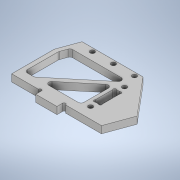
# Autodesk Inventor part: Trunk_lower_side_frame
Saved by Autodesk Inventor 2020.4 (Build 244396000, 396)
## iProperties
Created: 2022-01-02
Part Number: Trunk_lower_side_frame
Material: 一般
Document SubType Name: Modeling
Designer: Masato Kubotera
Density: 1 g/cm^3
Appearance: 既定
Mass: 14.6824 g
Surface Area: 92.1199 cm^2
Volume: 14.6824 cm^3
Description: A2017 T5
Author: Masato Kubotera
Autodesk Inventor part; units mm, degrees
ref_plane "YZ Plane" through (0, 0, 0) normal (1, 0, 0) x (0, 1, 0)
ref_plane "XZ Plane" through (0, 0, 0) normal (0, 1, 0) x (-1, 0, 0)
ref_plane "XY Plane" through (0, 0, 0) normal (0, 0, 1) x (1, 0, 0)
derived "Trunk_basis.ipt"
sketch "スケッチ1" plane through (0, 0, 0) normal (0, 1, 0) x (-1, 0, 0)
  line L0 (0, 22) -> (0, -143) construction
  circle A0 centre (5, 0) radius 10.5 construction
  line L1 (-7, 16) -> (36, 16) construction
  line L2 (36, 16) -> (36, -16) construction
  line L3 (36, -16) -> (-7, -16) construction
  line L4 (-7, -16) -> (-7, 16) construction
  line L5 (-7, 16) -> (36, -16) construction
  line L6 (36, 16) -> (-7, -16) construction
  line L7 (33, 13.5) -> (6, 13.5) construction
  line L8 (6, 13.5) -> (6, -13.5) construction
  line L9 (6, -13.5) -> (33, -13.5) construction
  line L10 (33, -13.5) -> (33, 13.5) construction
  line L11 (33, 13.5) -> (6, -13.5) construction
  line L12 (6, 13.5) -> (33, -13.5) construction
  line L13 (-7, 0) -> (36, 0) construction
  arc A1 (5, 16) -> (-7, 10.583) centre (5, 0) ccw construction
  line L14 (34.5651, -16.05) -> (5, -16.05) projected
  line L15 (5, 16.05) -> (34.5651, 16.05) projected
  line L16 (36.05, 14.5651) -> (36.05, -14.5651) projected
  line L17 (36.05, -16.05) -> (-7.05, 16.05) construction
  line L18 (-7.05, -16.05) -> (36.05, 16.05) construction
  arc A2 (5, 16.05) -> (-6.5314, 11.1638) centre (5, 0) ccw projected
  arc A3 (-6.5314, 11.1638) -> (-7.05, 9.8372) centre (-6.0721, 10.2196) ccw projected
  arc A4 (36.05, 14.5651) -> (34.5651, 16.05) centre (35.3075, 15.3075) ccw projected
  circle A5 centre (6, 13.5) radius 1.35 construction
  line L19 (19.5, 13.5) -> (19.5, -13.5) construction
  circle A6 centre (33, 13.5) radius 1.35 construction
  line L20 (-12, 22) -> (-17, 17) projected
  line L21 (-17, 17) -> (-17, -16) projected
  line L22 (-17, -16) -> (-28.5, -27.5) projected
  line L23 (-28.5, -27.5) -> (-28.5, -97) projected
  line L24 (54.5, -16) -> (54.5, 17) projected
  line L25 (54.5, 17) -> (49.5, 22) projected
  line L26 (49.5, 22) -> (-12, 22) projected
  line L27 (-28.5, -108.8772) -> (-28.5, -139) projected
  line L28 (-16, -138.9955) -> (-16, -99.5) construction
  line L29 (-16, -99.5) -> (16, -99.5) construction
  line L30 (16, -138.9955) -> (16, -99.5) construction
  line L31 (-7.5, -139) -> (-7.5, -143) projected
  line L32 (-7.5, -143) -> (7.5, -143) projected
  line L33 (7.5, -139) -> (7.5, -143) projected
  arc A7 (-7.5, -139) -> (-9.6, -139) centre (-8.55, -139) ccw projected
  arc A8 (9.6, -139) -> (7.5, -139) centre (8.55, -139) ccw projected
  line L34 (-22, -138.9955) -> (-22, -133) construction
  line L35 (-23.5, -133) -> (-20.5, -133) construction
  line L36 (-23.5, -133) -> (-23.5, -139) construction
  line L37 (-20.5, -133) -> (-20.5, -139) construction
  line L38 (-12, 22) -> (-7, 22) construction
  line L39 (-7, 22) -> (-7, -22) construction
  line L40 (-7, -22) -> (-12, -22) construction
  line L41 (-12, -22) -> (-12, 22) construction
  line L42 (-12, 22) -> (-7, -22) construction
  line L43 (-7, 22) -> (-12, -22) construction
  line L44 (-9.5, 22) -> (-9.5, -22) construction
  line L45 (-7, 0) -> (-12, 0) construction
  circle A9 centre (-9.5, 17.75) radius 1.6 projected
  line L46 (-12, 10) -> (-9.5, 10) construction
  line L47 (-9.5, 10) -> (-9.5, -10) construction
  line L48 (-9.5, -10) -> (-12, -10) construction
  line L49 (-12, -10) -> (-12, 10) construction
  line L50 (-12, 10) -> (-9.5, -10) construction
  line L51 (-9.5, 10) -> (-12, -10) construction
  line L52 (-9.45, 10.05) -> (-12.05, 10.05) projected
  line L53 (-12.05, 7.95) -> (-12.05, -7.95) projected
  line L54 (-12.05, -10.05) -> (-9.45, -10.05) projected
  line L55 (-9.45, -7.95) -> (-9.45, 7.95) projected
  line L56 (-9.45, 10.05) -> (-12.05, -10.05) construction
  line L57 (-12.05, 10.05) -> (-9.45, -10.05) construction
  arc A10 (-12.05, 10.05) -> (-12.05, 7.95) centre (-12.05, 9) ccw projected
  line L58 (-10.75, 10) -> (-10.75, -10) construction
  arc A11 (-9.45, 7.95) -> (-9.45, 10.05) centre (-9.45, 9) ccw projected
  circle A12 centre (-9.5, -17.75) radius 1.6 projected
  arc A13 (-12.05, -7.95) -> (-12.05, -10.05) centre (-12.05, -9) ccw projected
  arc A14 (-9.45, -10.05) -> (-9.45, -7.95) centre (-9.45, -9) ccw projected
  line L59 (36, 14.4) -> (44.5, 14.4) construction
  line L60 (44.5, 14.4) -> (44.5, -14.4) construction
  line L61 (36, -14.4) -> (44.5, -14.4) construction
  line L62 (46.95, 7.95) -> (46.95, -7.95) projected
  line L63 (49.5, 0) -> (44.5, 0) construction
  line L64 (44.5, 22) -> (49.5, 22) construction
  line L65 (49.55, -7.95) -> (49.55, 7.95) projected
  line L66 (48.25, 10) -> (48.25, -10) construction
  line L67 (49.5, 10) -> (47, -10) construction
  line L68 (49.5, -10) -> (47, -10) construction
  line L69 (49.5, 10) -> (49.5, -10) construction
  line L70 (47, 10) -> (49.5, -10) construction
  line L71 (46.95, -10.05) -> (49.55, -10.05) projected
  line L72 (46.95, 10.05) -> (49.55, -10.05) construction
  line L73 (49.55, 10.05) -> (46.95, -10.05) construction
  line L74 (49.5, -22) -> (44.5, -22) construction
  line L75 (44.5, 22) -> (49.5, -22) construction
  line L76 (49.5, 22) -> (49.5, -22) construction
  line L77 (49.5, 22) -> (44.5, -22) construction
  line L78 (47, 22) -> (47, -22) construction
  line L79 (44.5, -22) -> (44.5, 22) construction
  circle A15 centre (47, -17.75) radius 1.6 projected
  arc A16 (49.55, -10.05) -> (49.55, -7.95) centre (49.55, -9) ccw projected
  line L80 (47, -10) -> (47, 10) construction
  arc A17 (46.95, -7.95) -> (46.95, -10.05) centre (46.95, -9) ccw projected
  arc A18 (46.95, 10.05) -> (46.95, 7.95) centre (46.95, 9) ccw projected
  arc A19 (49.55, 7.95) -> (49.55, 10.05) centre (49.55, 9) ccw projected
  line L81 (47, 10) -> (49.5, 10) construction
  line L82 (49.55, 10.05) -> (46.95, 10.05) projected
  circle A20 centre (47, 17.75) radius 1.6 projected
  circle A21 centre (5, 0) radius 16 construction
  arc A22 (-6.5314, -11.1638) -> (5, -16.05) centre (5, 0) ccw projected
  arc A23 (-7.05, -9.8372) -> (-6.5314, -11.1638) centre (-6.0721, -10.2196) ccw projected
  arc A24 (34.5651, -16.05) -> (36.05, -14.5651) centre (35.3075, -15.3075) ccw projected
  line L83 (-7.05, -9.8372) -> (-7.05, 9.8372) projected
  line L84 (22, -138.9955) -> (22, -133) construction
  line L85 (23.5, -133) -> (23.5, -139) construction
  line L86 (20.5, -133) -> (20.5, -139) construction
  line L87 (23.5, -133) -> (20.5, -133) construction
  circle A25 centre (6, -13.5) radius 1.35 projected
  circle A26 centre (33, -13.5) radius 1.35 projected
  line L88 (188, -110.7642) -> (183, -110.7642) projected
  line L89 (183, -110.7642) -> (183, -167.2358) construction
  line L90 (183, -167.2358) -> (188, -167.2358) construction
  line L91 (188, -167.2358) -> (188, -110.7642) projected
  line L92 (188, -110.7642) -> (183, -167.2358) construction
  line L93 (183, -110.7642) -> (188, -167.2358) construction
  line L94 (22, -108.5) -> (56, -108.5) construction
  line L95 (56, -108.5) -> (56, -131.5) construction
  line L96 (56, -131.5) -> (22, -131.5) construction
  line L97 (22, -131.5) -> (22, -108.5) construction
  line L98 (22, -108.5) -> (56, -131.5) construction
  line L99 (56, -108.5) -> (22, -131.5) construction
  line L100 (22, -131.5) -> (52, -131.5) construction
  line L101 (52, -131.5) -> (52, -136.5) construction
  line L102 (52, -136.5) -> (22, -136.5) construction
  line L103 (22, -136.5) -> (22, -131.5) construction
  line L104 (22, -131.5) -> (52, -136.5) construction
  line L105 (52, -131.5) -> (22, -136.5) construction
  line L106 (-25.5, -131) -> (-25.5, -109.2298) projected
  line L107 (-8.2765, -133) -> (12.5, -133) projected
  line L108 (11.2211, -112.1814) -> (-9.5554, -129.4624) projected
  line L109 (22, -99.5) -> (17, -99.5) construction
  line L110 (17, -99.5) -> (17, -139) construction
  line L111 (17, -139) -> (22, -139) construction
  line L112 (22, -139) -> (22, -99.5) construction
  line L113 (22, -99.5) -> (17, -139) construction
  line L114 (17, -99.5) -> (22, -139) construction
  line L115 (19.5, -99.5) -> (19.5, -139) construction
  circle A27 centre (19.5, -107.25) radius 1.6 projected
  line L116 (17, -119.25) -> (22, -119.25) construction
  line L117 (-28.5, -139) -> (-28.5, -143) construction
  line L118 (-28.5, -143) -> (-7.5, -143) construction
  line L119 (28.5, -143) -> (7.5, -143) construction
  line L120 (28.5, -139) -> (28.5, -143) construction
  circle A28 centre (19.5, -131.25) radius 1.6 projected
  line L121 (17, -111.75) -> (22, -111.75) construction
  line L122 (17, -126.75) -> (22, -126.75) construction
  line L123 (39.4409, -150.6176) -> (61.7571, -150.6176) projected
  line L124 (63.242, -152.1025) -> (63.242, -179.9354) projected
  line L125 (61.7571, -181.4204) -> (39.4409, -181.4204) projected
  line L126 (37.9559, -179.9354) -> (37.9559, -152.1025) projected
  line L127 (37.9559, -150.6176) -> (63.242, -181.4204) construction
  line L128 (63.242, -150.6176) -> (37.9559, -181.4204) construction
  arc A29 (39.4409, -150.6176) -> (37.9559, -152.1025) centre (38.6984, -151.36) ccw projected
  line L129 (50.599, -150.6176) -> (50.599, -181.4204) construction
  line L130 (37.9559, -166.019) -> (63.242, -166.019) construction
  arc A30 (63.242, -152.1025) -> (61.7571, -150.6176) centre (62.4995, -151.36) ccw projected
  arc A31 (37.9559, -179.9354) -> (39.4409, -181.4204) centre (38.6984, -180.6779) ccw projected
  arc A32 (61.7571, -181.4204) -> (63.242, -179.9354) centre (62.4995, -180.6779) ccw projected
  arc A33 (18.4349, -111.7) -> (16.95, -113.1849) centre (17.6925, -112.4425) ccw projected
  line L131 (18.4349, -111.7) -> (20.5651, -111.7) projected
  arc A34 (22.05, -113.1849) -> (20.5651, -111.7) centre (21.3075, -112.4425) ccw projected
  line L132 (16.95, -125.3151) -> (16.95, -113.1849) projected
  line L133 (16.95, -119.25) -> (22.05, -119.25) construction
  arc A35 (16.95, -125.3151) -> (18.4349, -126.8) centre (17.6925, -126.0575) ccw projected
  line L134 (19.5, -111.7) -> (19.5, -126.8) construction
  line L135 (16.95, -111.7) -> (22.05, -126.8) construction
  line L136 (22.05, -111.7) -> (16.95, -126.8) construction
  line L137 (20.5651, -126.8) -> (18.4349, -126.8) projected
  line L138 (22.05, -113.1849) -> (22.05, -125.3151) projected
  arc A36 (20.5651, -126.8) -> (22.05, -125.3151) centre (21.3075, -126.0575) ccw projected
  line L139 (37, -131.5) -> (37, -136.5) construction
  line L140 (32, -131.5) -> (32, -136.5) construction
  line L141 (52, -134) -> (22, -134) projected
  circle A37 centre (27, -134) radius 1.6 projected
  arc A38 (42.05, -132.9349) -> (40.5651, -131.45) centre (41.3075, -132.1925) ccw projected
  arc A39 (33.4349, -131.45) -> (31.95, -132.9349) centre (32.6925, -132.1925) ccw projected
  line L142 (31.95, -134) -> (42.05, -134) construction
  line L143 (33.4349, -131.45) -> (40.5651, -131.45) projected
  line L144 (42.05, -132.9349) -> (42.05, -135.0651) projected
  line L145 (40.5651, -136.55) -> (33.4349, -136.55) projected
  line L146 (31.95, -135.0651) -> (31.95, -132.9349) projected
  line L147 (31.95, -131.45) -> (42.05, -136.55) construction
  line L148 (42.05, -131.45) -> (31.95, -136.55) construction
  line L149 (37, -131.45) -> (37, -136.55) construction
  arc A40 (31.95, -135.0651) -> (33.4349, -136.55) centre (32.6925, -135.8075) ccw projected
  arc A41 (40.5651, -136.55) -> (42.05, -135.0651) centre (41.3075, -135.8075) ccw projected
  line L150 (42, -131.5) -> (42, -136.5) construction
  circle A42 centre (47, -134) radius 1.6 projected
  line L151 (-23.6994, -103.9301) -> (-25.3794, -108.5458) projected
  line L152 (-23.5, -133) -> (-19.223, -133) projected
  line L153 (-17.9441, -132.5376) -> (13.7789, -106.1518) projected
  line L154 (-23.5, -22.5) -> (61, -22.5) construction
  line L155 (54.5, -16) -> (61, -22.5) projected
  line L156 (61, -22.5) -> (61, -89.4955) projected
  circle A43 centre (-13.5, -55) radius 1.75 projected
  line L157 (-16.5, -59) -> (49, -59) projected
  line L158 (51, -61) -> (51, -87.5) projected
  line L159 (49, -89.5) -> (-16.5, -89.5) projected
  line L160 (-18.5, -87.5) -> (-18.5, -61) projected
  line L161 (-18.5, -59) -> (51, -89.5) construction
  line L162 (51, -59) -> (-18.5, -89.5) construction
  line L163 (-16.5, -27.5) -> (49, -27.5) projected
  line L164 (51, -29.5) -> (51, -49) projected
  line L165 (49, -51) -> (-16.5, -51) projected
  line L166 (-18.5, -49) -> (-18.5, -29.5) projected
  line L167 (-18.5, -27.5) -> (51, -51) construction
  line L168 (51, -27.5) -> (-18.5, -51) construction
  line L169 (-23.5, -102) -> (-28.5, -97) projected
  line L170 (-23.5, -99.5) -> (56, -99.5) construction
  line L171 (56, -99.5) -> (56, -94.5) construction
  line L172 (56, -94.5) -> (-23.5, -94.5) construction
  line L173 (-23.5, -94.5) -> (-23.5, -99.5) construction
  line L174 (-23.5, -99.5) -> (56, -94.5) construction
  line L175 (56, -99.5) -> (-23.5, -94.5) construction
  line L176 (-23.5, -97) -> (56, -97) construction
  line L177 (16.25, -94.5) -> (16.25, -99.5) construction
  circle A44 centre (-13.496, -97) radius 1.6 projected
  circle A45 centre (1.377, -97) radius 1.6 projected
  circle A46 centre (16.25, -97) radius 1.6 projected
  circle A47 centre (31.123, -97) radius 1.6 projected
  circle A48 centre (45.996, -97) radius 1.6 projected
  line L178 (14.5, -113.7191) -> (14.5, -131) projected
  line L179 (16.5, -139) -> (61, -139) projected
  line L180 (61, -139) -> (61, -94.4955) projected
  line L181 (-28.5, -139) -> (-9.6, -139) projected
  line L182 (9.6, -139) -> (28.5, -139) projected
  line L183 (-23.2671, -94.5) -> (19.7825, -94.5) projected
  line L184 (19.7825, -94.5) -> (41.662, -120.575) projected
  line L185 (41.662, -120.575) -> (33.5, -143) projected
  line L186 (33.5, -143) -> (28.55, -143) projected
  line L187 (28.55, -139) -> (28.55, -143) projected
  line L188 (-23.2671, -94.5) -> (-28.5, -108.8772) projected
  line L189 (61, -89.4955) -> (61, -94.4955) projected
  arc A49 (-16.5, -27.5) -> (-18.5, -29.5) centre (-16.5, -29.5) ccw projected
  arc A50 (-18.5, -49) -> (-16.5, -51) centre (-16.5, -49) ccw projected
  arc A51 (49, -51) -> (51, -49) centre (49, -49) ccw projected
  arc A52 (51, -29.5) -> (49, -27.5) centre (49, -29.5) ccw projected
  arc A53 (-16.5, -59) -> (-18.5, -61) centre (-16.5, -61) ccw projected
  arc A54 (-18.5, -87.5) -> (-16.5, -89.5) centre (-16.5, -87.5) ccw projected
  arc A55 (49, -89.5) -> (51, -87.5) centre (49, -87.5) ccw projected
  arc A56 (51, -61) -> (49, -59) centre (49, -61) ccw projected
  line L190 (-28.5, -108.8772) -> (-25.5, -108.8772) construction
  arc A57 (14.5, -137) -> (16.5, -139) centre (16.5, -137) ccw projected
  arc A58 (14.5, -104.6142) -> (12.5, -102.6142) centre (12.5, -104.6142) ccw projected
  arc A59 (13.7789, -106.1518) -> (14.5, -104.6142) centre (12.5, -104.6142) ccw projected
  arc A60 (-21.82, -102.6142) -> (-23.6994, -103.9301) centre (-21.82, -104.6142) ccw projected
  arc A61 (-19.223, -133) -> (-17.9441, -132.5376) centre (-19.223, -131) ccw projected
  arc A62 (-25.5, -131) -> (-23.5, -133) centre (-23.5, -131) ccw projected
  arc A63 (-25.3794, -108.5458) -> (-25.5, -109.2298) centre (-23.5, -109.2298) ccw projected
  arc A64 (-9.5554, -129.4624) -> (-8.2765, -133) centre (-8.2765, -131) ccw projected
  arc A65 (12.5, -133) -> (14.5, -131) centre (12.5, -131) ccw projected
  arc A66 (14.5, -113.7191) -> (11.2211, -112.1814) centre (12.5, -113.7191) ccw projected
  line L191 (-21.82, -102.6142) -> (12.5, -102.6142) projected
  line L192 (-23.5, -102) -> (14.5, -102) projected
  line L193 (14.5, -102) -> (14.5, -137) projected
  point P0 (0, 0)
  point P1 (14.5, 0)
  point P2 (19.5, 0)
  point P3 (-7.05, 10.6019)
  point P4 (19.5, 0)
  point P5 (-9.5, 0)
  point P6 (-10.75, 0)
  point P7 (36.05, 14.4)
  point P8 (36.05, -14.4)
  point P9 (48.25, 0)
  point P10 (47, 0)
  point P11 (185.5, -139)
  point P12 (39, -120)
  point P13 (37, -134)
  point P14 (-25.5, -133)
  point P15 (-13.5728, -133)
  point P16 (19.5, -119.25)
  point P17 (50.599, -166.019)
  point P18 (19.5, -119.25)
  point P19 (19.5, -119.25)
  point P20 (37, -134)
  point P21 (37, -134)
  point P22 (-18.5, -133)
  point P23 (16.25, -74.25)
  point P24 (16.25, -39.25)
  point P25 (30.6126, -98.1486)
  point P26 (27.8987, -96.9989)
  point P27 (37.7039, -131.45)
  point P28 (34.9559, -139)
  point P29 (35.8476, -136.55)
  dimension "d4" = 44
  measures "d4" distance of L84.start L34.start
extrude "押し出し1" add sketch "スケッチ1" along normal blind 5 contours L188 L183 L184 L185 L143 A39 L146 A40 L145 L179 A57 L193 L178 L192 L169 | L169 L192 L193 A66 L108 A64 L107 A65 A57 L182 A8 L33 L32 L31 A7 L181 L27 L188 | L185 L141 L146 A39 L143 | L145 A40 L146 L141 L185 | A37 L141 | L141 A37
